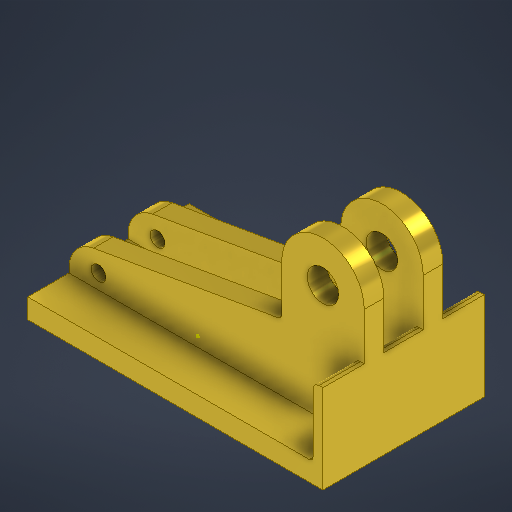
# Autodesk Inventor part: Part1
Saved by Autodesk Inventor 2026.2 (Build 302298000, 298)
## iProperties
Created: 2026-03-24
Part Number: Part1
Material: Generic
Document SubType Name: Modeling
Designer: LENOVO
Density: 1 g/cm^3
Appearance: Metal 2400F Hot
Author: LENOVO
Autodesk Inventor part; units mm, degrees
ref_plane "YZ Plane" through (0, 0, 0) normal (1, 0, 0) x (0, 1, 0)
ref_plane "XZ Plane" through (0, 0, 0) normal (0, 1, 0) x (-1, 0, 0)
sketch "Sketch1" plane through (0, 0, 0) normal (0, 0, 1) x (1, 0, 0)
  line L0 (79.3694, 29.7923) -> (84.3694, 29.7923)
  line L1 (84.3694, 29.7923) -> (84.3694, -15.2077)
  line L2 (84.3694, -15.2077) -> (-65.6306, -15.2077)
  line L3 (-65.6306, -15.2077) -> (-65.6306, -5.2077)
  line L4 (-65.6306, -5.2077) -> (79.3694, -5.2077)
  line L5 (79.3694, -5.2077) -> (79.3694, 29.7923)
  line L6 (79.3694, 29.7923) -> (84.3694, 29.7923)
  point P0 (0, 0)
  dimension "d0" = 45
  dimension "d1" = 150
  dimension "d2" = 10
  dimension "d3" = 5
  constraints: 14 end point, 3 perpendicular, 1 collinear, 1 horizontal
  measures "d0" distance of L0.end L1.end
  measures "d1" distance of L1.end L2.end
  measures "d2" distance of L2.end L3.end
  measures "d3" distance of L0.start L0.end
extrude "Extrusion1" add sketch "Sketch1" against normal blind 82
fillet "Fillet1" radius 3 1 edges at (79.3694, 29.7923, -41)
fillet "Fillet2" radius 2 1 edges at (79.3694, -5.2077, -41)
ref_plane "Work Plane1" through (0, 0, -21) normal (0, 0, 1) x (1, 0, 0)
sketch "Sketch2" plane through (0, 0, -21) normal (0, 0, 1) x (1, 0, 0)
  point P0 (0, 0)
sketch "Sketch3" plane through (0, 0, -21) normal (0, 0, 1) x (1, 0, 0)
  line L0 (-65.6306, -15.2077) -> (-65.6306, -5.2077) projected
  line L1 (-65.6306, -5.2077) -> (-65.6306, 9.7923)
  line L2 (-65.6306, 9.7923) -> (42.3694, 28.5423)
  line L3 (-65.6306, -5.2077) -> (77.3694, -5.2077) projected
  line L4 (54.3694, -5.2077) -> (84.3564, -5.2077)
  arc A0 (77.3694, -5.2077) -> (79.3694, -3.2077) centre (77.3694, -3.2077) ccw projected
  line L5 (77.3694, -5.2077) -> (79.3694, -3.2077)
  line L6 (79.3694, -3.2077) -> (79.3694, 26.9279)
  line L7 (79.3694, 26.9279) -> (81.3477, 29.7923)
  line L8 (81.3477, 29.7923) -> (82.0785, 29.7923)
  line L9 (82.3694, 29.7923) -> (84.3694, 29.7923) projected
  line L10 (82.0785, 29.7923) -> (84.3694, 29.7923)
  line L11 (84.3694, 29.7923) -> (84.3694, 74.7923)
  line L12 (84.3694, 74.7923) -> (42.3694, 74.7923)
  line L13 (42.3694, 74.7923) -> (42.3694, 28.5423)
  point P0 (0, 0)
  point P1 (77.3694, -5.2077)
  dimension "d9" = 15
  dimension "d12" = 108
  dimension "d13" = 25
  dimension "d21" = 45
  dimension "d23" = 42
  constraints: 22 end point, 3 perpendicular, 2 horizontal, 2 vertical, 1 collinear, 1 point on line, 1 tangent
  measures "d9" distance of L0.end L1.end
  measures "d12" horizontal distance of L1.end L2.end
  measures "d13" distance of L0.start L1.end
  measures "d21" distance of L9.end L11.end
  measures "d23" distance of L11.end L12.end
extrude "Extrusion2" add sketch "Sketch3" against normal blind 10 contours L1 L2 L13 L12 L11 L9 L10 L8 L7 L6 L5 L3
fillet "Fillet4" radius 21 2 edges at (84.3694, 74.7923, -26) (42.3694, 74.7923, -26)
fillet "Fillet5" radius 15 1 edges at (-65.6306, 9.7923, -26)
sketch "Sketch4" plane through (0, 0, -21) normal (0, 0, 1) x (1, 0, 0)
  point P0 (0, 0)
ref_plane "Work Plane3" through (0, 0, -51) normal (0, 0, 1) x (1, 0, 0)
sketch "Sketch6" plane through (0, 0, -51) normal (0, 0, 1) x (1, 0, 0)
  line L0 (77.3694, -5.2077) -> (-65.6306, -5.2077) projected
  arc A0 (-53.1963, 11.951) -> (-65.6306, -2.8279) centre (-50.6306, -2.8279) ccw projected
  line L1 (-65.6306, -2.8279) -> (-65.6306, -5.2077) projected
  line L2 (77.3694, -5.2077) -> (-65.6306, -5.2077) projected
  line L3 (77.3694, -5.2077) -> (79.3694, -3.2077) projected
  line L4 (79.3694, 26.7923) -> (79.3694, -3.2077) projected
  line L5 (79.3694, 26.7923) -> (79.3694, 26.9279) projected
  line L6 (79.3694, 26.9279) -> (79.3727, 26.9326) projected
  arc A1 (81.1769, 29.5451) -> (79.3727, 26.9326) centre (82.3694, 26.7923) ccw projected
  line L7 (81.1769, 29.5451) -> (81.3477, 29.7923) projected
  line L8 (81.3477, 29.7923) -> (82.3694, 29.7923) projected
  line L9 (84.3694, 29.7923) -> (82.3694, 29.7923) projected
  line L10 (84.3694, 29.7923) -> (84.3694, 53.7923) projected
  arc A2 (84.3694, 53.7923) -> (42.3694, 53.7923) centre (63.3694, 53.7923) ccw projected
  line L11 (42.3694, 53.7923) -> (42.3694, 28.5423) projected
  line L12 (42.3694, 28.5423) -> (-53.1963, 11.951) projected
  point P0 (0, 0)
extrude "Extrusion3" add sketch "Sketch6" against normal blind 10
sketch "Sketch7" plane through (0, 0, -21) normal (0, 0, 1) x (1, 0, 0)
  line L0 (-65.6306, -5.2077) -> (77.3694, -5.2077) projected
  line L1 (-65.6306, -5.2077) -> (77.3694, -5.2077) projected
  line L2 (-53.1963, 11.951) -> (42.3694, 28.5423) projected
  arc A0 (-53.1963, 11.951) -> (-65.6306, -2.8279) centre (-50.6306, -2.8279) ccw projected
  circle A1 centre (-50.6306, 2.2923) radius 3.75
  line L3 (42.3694, 53.7923) -> (42.3694, 28.5423) projected
  arc A2 (84.3694, 53.7923) -> (42.3694, 53.7923) centre (63.3694, 53.7923) ccw projected
  circle A3 centre (63.3694, 53.7923) radius 8
  point P0 (0, 0)
  point P1 (-50.6306, -5.2077)
  dimension "d29" = 15
  dimension "d30" = 7.5
  dimension "d31" = 7.5
  dimension "d34" = 16
  constraints: 3 coincident, 2 centre point, 1 point on line
  measures "d29" distance of point (-65.631, -5.208) point (-50.631, -5.208)
  measures "d30" distance of point (-50.631, -5.208) point (-50.631, 2.292)
  measures "d31" diameter of A1
  measures "d34" diameter of A3
extrude "Extrusion4" cut sketch "Sketch7" against normal blind 40 contours A1
sketch "Sketch8" plane through (0, 0, -21) normal (0, 0, 1) x (1, 0, 0)
  arc A0 (84.3694, 53.7923) -> (42.3694, 53.7923) centre (63.3694, 53.7923) ccw projected
  circle A1 centre (63.3694, 53.7923) radius 8
  point P0 (0, 0)
  dimension "d35" = 16
  constraints: 1 centre point, 1 coincident
  measures "d35" diameter of A1
extrude "Extrusion5" cut sketch "Sketch8" against normal blind 40
fillet "Fillet6" radius 2 2 edges at (42.3694, 28.5423, -26) (42.3694, 28.5423, -56)
body "Solid1"
